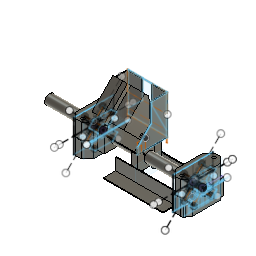
x-y-axis-on-pipe (Autodesk Fusion 360 design; units mm, degrees)
Autodesk Fusion 360 part; units mm, degrees
sketch "Sketch1" plane through (0, 0, 0) normal (1, 0, 0) x (0, 1, 0) in component "pipe-d25mm"
  circle A0 centre (0, 0) radius 12.5
  circle A1 centre (0, 0) radius 11
  dimension "d1" = 25
  dimension "d4" = 22
  constraint coincident A0.centre A1.centre
  constraint concentric A0 A1
  measures "d1" diameter of A0
  measures "d4" diameter of A1
extrude "Extrude1" add sketch "Sketch1" against normal blind 395 makes body 1 in component "pipe-d25mm"
sketch "Sketch1 (2)" plane through (0, 0, 0) normal (1, 0, 0) x (0, 1, 0) in component "pipe-slider"
  circle A0 centre (0, 0) radius 11
  circle A1 centre (0, 0) radius 12.5
  line L0 (0, 0) -> (50, 0) construction
  line L1 (50, 0) -> (50, -40) construction
  line L2 (50, -40) -> (0, -40) construction
  line L3 (0, -40) -> (0, 0) construction
  line L4 (50, 0) -> (-50, 0)
  line L5 (-50, 0) -> (-50, -40)
  line L6 (-50, -40) -> (50, -40)
  line L7 (50, -40) -> (50, 0)
  line L8 (0, 0) -> (61.3417, -61.3417) construction
  line L9 (0, 0) -> (86.7503, 0) construction
  line L10 (0, 0) -> (-70.1783, -70.1783) construction
  line L11 (0, 0) -> (99.2472, 0) construction
  line L12 (8.8388, -8.8388) -> (24.3952, -24.3952) construction
  line L13 (8.8388, -8.8388) -> (16.617, -16.617) construction
  line L14 (-8.8388, -8.8388) -> (-16.617, -16.617) construction
  line L15 (8.8388, -8.8388) -> (24.3952, -24.3952) construction
  line L16 (24.3952, -24.3952) -> (27.9307, -20.8597) construction
  line L17 (27.9307, -20.8597) -> (12.3744, -5.3033) construction
  line L18 (12.3744, -5.3033) -> (8.8388, -8.8388) construction
  line L19 (-8.8388, -8.8388) -> (-24.3952, -24.3952) construction
  line L20 (-24.3952, -24.3952) -> (-27.9307, -20.8597) construction
  line L21 (-27.9307, -20.8597) -> (-12.3744, -5.3033) construction
  line L22 (12.3744, -5.3033) -> (5.3033, -12.3744) construction
  line L23 (5.3033, -12.3744) -> (22.2739, -29.3449) construction
  line L24 (22.2739, -29.3449) -> (29.3449, -22.2739) construction
  line L25 (29.3449, -22.2739) -> (12.3744, -5.3033) construction
  line L26 (-5.3033, -12.3744) -> (-22.2739, -29.3449) construction
  line L27 (-22.2739, -29.3449) -> (-29.3449, -22.2739) construction
  line L28 (-29.3449, -22.2739) -> (-12.3744, -5.3033) construction
  line L29 (29.3449, -22.2739) -> (22.2739, -29.3449)
  line L30 (4, 0) -> (5.5355, 1.5355)
  circle A2 centre (0, 0) radius 13.5
  line L31 (22.2739, -29.3449) -> (5.3033, -12.3744)
  line L32 (12.3744, -5.3033) -> (29.3449, -22.2739)
  line L33 (-5.3033, -12.3744) -> (-22.2739, -29.3449)
  line L34 (-22.2739, -29.3449) -> (-29.3449, -22.2739)
  line L35 (-29.3449, -22.2739) -> (-12.3744, -5.3033)
  dimension "d5" = 50
  dimension "d6" = 40
  dimension "d7" = 100
  dimension "d8" = 45
  dimension "d9" = 135
  dimension "d10" = 22
  dimension "d11" = 11
  dimension "d12" = 11
  dimension "d13" = 5
  dimension "d14" = 22
  dimension "d15" = 5
  dimension "d16" = 10
  dimension "d17" = 24
  dimension "d18" = 10
  dimension "d19" = 24
  dimension "d20" = 27
  dimension "d21" = 24
  constraint horizontal L0
  constraint vertical L1
  constraint horizontal L2
  constraint vertical L3
  constraint coincident A0.centre A1.centre
  constraint horizontal L4
  constraint vertical L5
  constraint horizontal L6
  constraint vertical L7
  constraint horizontal L9
  constraint horizontal L11
  constraint coincident L8 L12.start
  constraint coincident A1 L12.start
  constraint parallel L8 L12
  constraint parallel L8 L13
  constraint coincident L10 L14.start
  constraint coincident A1 L14.start
  constraint perpendicular L13 L14
  constraint perpendicular L15 L16
  constraint parallel L15 L17
  constraint parallel L16 L18
  constraint perpendicular L19 L20
  constraint parallel L19 L21
  constraint coincident L10 L19.end
  constraint perpendicular L22 L23
  constraint parallel L22 L24
  constraint parallel L23 L25
  constraint perpendicular L12 L22
  constraint parallel L26 L28
  constraint perpendicular L29 L31
  constraint parallel L29 L30
  constraint coincident L0 L30.start
  constraint parallel L33 L35
  measures "d5" distance of A0.centre L0.end
  measures "d6" distance of A0.centre L2.end
  measures "d7" distance of L0.end L4.end
  measures "d8" angle of L8 L9
  measures "d9" angle of L10 L11
  measures "d10" distance of L12.start L12.end
  measures "d11" distance of L12.start L13.end
  measures "d12" distance of L14.start L14.end
  measures "d13" distance of L12.start L17.end
  measures "d14" distance of L14.start L19.end
  measures "d15" distance of L14.start L21.end
  measures "d16" distance of L17.end L22.end
  measures "d17" distance of L17.end L24.end
  measures "d18" distance of L21.end L26.start
  measures "d19" distance of L21.end L27.end
  measures "d20" diameter of A2
  measures "d21" distance of L21.end L27.end
extrude "Extrude7" add sketch "Sketch1 (2)" against normal blind 10 separate body contours L4 L5 L6 L7 L29 A2 L31 L32 L33 L34 L35 | L29 A2 L31 L32 | A2 L33 L34 L35 makes body 2 in component "pipe-slider"
extrude "Extrude1'" add sketch "Sketch1 (2)" along normal blind 24 separate body contours L4 L5 L6 L7 L29 A2 L31 L32 L33 L34 L35 makes body 3 in component "pipe-slider"
sketch "Sketch2" plane through (24, 0, 0) normal (1, 0, 0) x (0, 1, 0) in component "pipe-slider"
  line L0 (-5.3315, -12.4026) -> (-22.2739, -29.3449)
  line L1 (-22.2739, -29.3449) -> (-29.3449, -22.2739)
  line L2 (-29.3449, -22.2739) -> (-12.4026, -5.3315)
  arc A0 (-13.5, 0) -> (-12.4026, -5.3315) centre (0, 0) ccw
  line L3 (-13.5, 0) -> (-50, 0)
  line L4 (-50, 0) -> (-50, -40)
  line L5 (-50, -40) -> (50, -40)
  line L6 (50, -40) -> (50, 0)
  line L7 (50, 0) -> (13.5, 0)
  arc A1 (12.4026, -5.3315) -> (13.5, 0) centre (0, 0) ccw
  line L8 (12.4026, -5.3315) -> (29.3449, -22.2739)
  line L9 (29.3449, -22.2739) -> (22.2739, -29.3449)
  line L10 (22.2739, -29.3449) -> (5.3315, -12.4026)
  arc A2 (-5.3315, -12.4026) -> (5.3315, -12.4026) centre (0, 0) ccw
sketch "Sketch3" plane through (0, 3.5355, -3.5355) normal (0, -0.707107, 0.707107) x (1, 0, 0) in component "pipe-slider"
  line L0 (0, -12.5399) -> (0, -36.5)
  line L1 (0, -36.5) -> (24, -36.5)
  line L2 (24, -36.5) -> (24, -12.5399)
  line L3 (24, -12.5399) -> (0, -12.5399)
  line L4 (0, -36.5) -> (24, -36.5) construction
  line L5 (24, -36.5) -> (24, -34.5) construction
  line L6 (24, -34.5) -> (0, -34.5) construction
  line L7 (0, -34.5) -> (0, -36.5) construction
  line L8 (0, -34.5) -> (1, -34.5) construction
  line L9 (1, -34.5) -> (1, -12.5) construction
  line L10 (1, -12.5) -> (0, -12.5) construction
  line L11 (0, -12.5) -> (0, -34.5) construction
  line L12 (1, -34.5) -> (1, -12.5) construction
  line L13 (1, -12.5) -> (23, -12.5) construction
  line L14 (23, -12.5) -> (23, -34.5) construction
  line L15 (23, -34.5) -> (1, -34.5) construction
  line L16 (1, -34.5) -> (23, -12.5) construction
  line L17 (23, -34.5) -> (1, -12.5) construction
  circle A0 centre (12, -23.5) radius 4
  dimension "d24" = 2
  dimension "d25" = 22
  dimension "d26" = 22
  dimension "d27" = 22
  dimension "d28" = 8
  constraint perpendicular L4 L5
  constraint parallel L4 L6
  constraint parallel L5 L7
  constraint coincident L1.end L2.start
  constraint perpendicular L2 L4
  constraint coincident L0.end L1.start
  constraint perpendicular L8 L9
  constraint parallel L8 L10
  constraint parallel L9 L11
  constraint coincident L6 L8.end
  constraint perpendicular L12 L13
  constraint parallel L12 L14
  constraint parallel L13 L15
  constraint perpendicular L3 L12
  constraint midpoint L17 A0.centre
  measures "d24" distance of L0.end L6.end
  measures "d25" distance of L6.end L10.end
  measures "d26" distance of L8.end L9.end
  measures "d27" distance of L8.end L14.end
  measures "d28" diameter of A0
extrude "Extrude3" cut sketch "Sketch3" along normal blind 38 contours A0 bodies 3 in component "pipe-slider"
extrude "Extrude2" cut sketch "Sketch3" against normal blind 10 contours A0 bodies 3 in component "pipe-slider"
sketch "Sketch4" plane through (0, -3.5355, -3.5355) normal (0, 0.707107, 0.707107) x (-1, 0, 0) in component "pipe-slider"
  line L0 (0, -36.5) -> (0, -12.5399)
  line L1 (0, -12.5399) -> (-24, -12.5399)
  line L2 (-24, -12.5399) -> (-24, -36.5)
  line L3 (-24, -36.5) -> (0, -36.5)
  line L4 (0, -36.5) -> (-24, -36.5) construction
  line L5 (-24, -36.5) -> (-24, -34.5) construction
  line L6 (-24, -34.5) -> (0, -34.5) construction
  line L7 (0, -34.5) -> (0, -36.5) construction
  line L8 (-24, -34.5) -> (-23, -34.5) construction
  line L9 (-23, -34.5) -> (-23, -12.5) construction
  line L10 (-23, -12.5) -> (-24, -12.5) construction
  line L11 (-24, -12.5) -> (-24, -34.5) construction
  line L12 (-23, -34.5) -> (-1, -34.5) construction
  line L13 (-1, -34.5) -> (-1, -12.5) construction
  line L14 (-1, -12.5) -> (-23, -12.5) construction
  line L15 (-23, -12.5) -> (-23, -34.5) construction
  line L16 (-1, -34.5) -> (-23, -12.5) construction
  line L17 (-23, -34.5) -> (-1, -12.5) construction
  circle A0 centre (-12, -23.5) radius 4
  dimension "d33" = 2
  dimension "d34" = 22
  dimension "d35" = 22
  dimension "d36" = 8
  constraint perpendicular L4 L5
  constraint parallel L4 L6
  constraint parallel L5 L7
  constraint coincident L2.end L3.start
  constraint perpendicular L2 L4
  constraint coincident L0.start L3.end
  constraint perpendicular L8 L9
  constraint parallel L8 L10
  constraint parallel L9 L11
  constraint coincident L6 L8.end
  constraint perpendicular L2 L8
  constraint perpendicular L12 L13
  constraint parallel L12 L14
  constraint parallel L13 L15
  constraint coincident L6 L12.end
  constraint midpoint L17 A0.centre
  measures "d33" distance of L0.start L6.end
  measures "d34" distance of L5.end L10.end
  measures "d35" distance of L8.end L9.end
  measures "d36" diameter of A0
extrude "Extrude5" cut sketch "Sketch4" along normal blind 45 contours A0 bodies 3 in component "pipe-slider"
extrude "Extrude4" cut sketch "Sketch4" against normal blind 10 contours A0 bodies 3 in component "pipe-slider"
sketch "Sketch1 (3)" plane through (0, -3.5355, -3.5355) normal (0, 0.707107, 0.707107) x (-1, 0, 0) in component "washer"
  circle A0 centre (-12, -23.5) radius 3.5
  circle A1 centre (-12, -23.5) radius 8
  dimension "d41" = 7
  dimension "d42" = 16
  constraint concentric A0 A1
  measures "d41" diameter of A0
  measures "d42" diameter of A1
extrude "Extrude1''" add sketch "Sketch1 (3)" along normal blind 1.5 separate body makes body 4 in component "washer"
sketch "Sketch1 (4)" plane through (0, -2.4749, -2.4749) normal (0, 0.707107, 0.707107) x (-1, 0, 0) in component "bearing8x22x7"
  circle A0 centre (-12, -23.5) radius 3.5
  circle A1 centre (-12, -23.5) radius 8
  circle A2 centre (-12, -23.5) radius 3.5
  circle A3 centre (-12, -23.5) radius 11
  dimension "d45" = 22
  constraint concentric A0 A2
  constraint concentric A2 A3
  measures "d45" diameter of A3
extrude "Extrude1'''" add sketch "Sketch1 (4)" along normal blind 7 separate body contours A1 | A3 makes body 5 in component "bearing8x22x7"
sketch "Sketch6" plane through (24, 0, 0) normal (1, 0, 0) x (0, 1, 0) in component "pipe-slider"
  arc A0 (-13.5, 0) -> (13.5, 0) centre (0, 0) ccw
  line L0 (-13.5, 0) -> (-33.4897, -23.065)
  line L1 (-33.4897, -23.065) -> (-19.8622, -34.8755)
  line L2 (-19.8622, -34.8755) -> (24.3662, -35.2868)
  line L3 (24.3662, -35.2868) -> (35.669, -22.2451)
  line L4 (35.669, -22.2451) -> (13.5, 0)
  constraint coincident A0.centre origin
  constraint perpendicular L0 L1
  constraint perpendicular L1 L3
extrude "Extrude6" add sketch "Sketch2" sketch "Sketch6" along normal blind 10 of sketch 2 bodies 3 in component "pipe-slider"
sketch "Sketch7" plane through (0, 0, 0) normal (0, 0, 1) x (-1, 0, 0) in component "pipe-slider"
  ellipse E0 centre (-12, -33.234) end of major axis (-12, -27.5772) minor radius 4
  line L0 (0, -50) -> (0, -13.5)
  line L1 (0, -13.5) -> (-34, -13.5)
  line L2 (-34, -13.5) -> (-34, -50)
  line L3 (-34, -50) -> (0, -50)
  circle A0 centre (-12.5, -40) radius 4
  circle A1 centre (-12.5, 40) radius 4
  dimension "d52" = 8
  dimension "d53" = 8
  measures "d52" diameter of A0
  measures "d53" diameter of A1
extrude "Extrude8" cut sketch "Sketch7" against normal blind 46 contours E0 A0 | E0 A0 | A1 picked at (-12.249, -36.9652) picked at (-12.4627, -42.2784) bodies 3 in component "pipe-slider"
combine "Combine1" operation add target body 2 tool bodies 3 in component "pipe-slider"
chamfer "Chamfer1" distance 15 angle 45 4 edges at (34, 50, -20) (34, -50, -20) (-10, -50, -20) (-10, 50, -20) on bodies 2 in component "pipe-slider"
sketch "Sketch8" plane through (34, 0, 0) normal (1, 0, 0) x (0, 1, 0) in component "pipe-slider"
  line L0 (-35, 0) -> (-35, -40)
  line L1 (-35, -40) -> (35, -40)
  line L2 (35, -40) -> (35, 0)
  line L3 (35, 0) -> (13.5, 0)
  arc A0 (-13.5, 0) -> (13.5, 0) centre (0, 0) ccw
  line L4 (-13.5, 0) -> (-35, 0)
  line L5 (-52, 1) -> (-52, -0.5)
  line L6 (-52, 1) -> (55.5207, 1)
  line L7 (55.5207, 1) -> (55.5207, -0.5)
  line L8 (55.5207, -0.5) -> (-52, -0.5)
  line L9 (-52, -0.5) -> (-52, 1)
  dimension "d57" = 1.5
  constraint vertical L5
  constraint horizontal L6
  constraint vertical L7
  constraint horizontal L8
  constraint vertical L9
  measures "d57" distance of L5.start L5.end
extrude "Extrude9" cut sketch "Sketch8" against normal blind 61 contours L0 A0 L4 L8 | L0 L2 L3 A0 L4 L5 L6 L7 L8 L9 | L2 L3 A0 L8 bodies 2 in component "pipe-slider"
sketch "Sketch1 (5)" plane through (0, -10.6066, -10.6066) normal (0, 0.707107, 0.707107) x (-1, 0, 0) in component "stud-30mm-d8mm"
  circle A0 centre (-12, -23.5) radius 4
extrude "Extrude1''''" add sketch "Sketch1 (5)" along normal blind 30 separate body makes body 6 in component "stud-30mm-d8mm"
sketch "Sketch1 (6)" plane through (-10, 0, 0) normal (-1, 0, 0) x (0, -1, 0) in component "frame-bottom"
  line L0 (35, -0.5) -> (13.4907, -0.5)
  arc A0 (-13.4907, -0.5) -> (13.4907, -0.5) centre (0, 0) ccw
  line L1 (-13.4907, -0.5) -> (-35, -0.5)
  line L2 (-35, -0.5) -> (-35, -40)
  line L3 (-35, -40) -> (35, -40)
  line L4 (35, -40) -> (35, -0.5)
  line L5 (30, 20) -> (-45, 20)
  line L6 (-45, 20) -> (-45, 118)
  line L7 (-45, 118) -> (-4, 118)
  line L8 (30, 35) -> (30, 20)
  line L9 (-45, 118) -> (-4, 118) construction
  line L10 (-45, 70) -> (-45, 118) construction
  line L11 (30, 20) -> (20, 20) construction
  line L12 (20, 20) -> (20, 35) construction
  line L13 (20, 35) -> (30, 35) construction
  line L14 (30, 35) -> (30, 20) construction
  line L15 (30, 35) -> (-4, 70)
  line L16 (-4, 118) -> (-4, 70)
  line L17 (30, 20) -> (10, 20) construction
  line L18 (10, 20) -> (10, 46) construction
  line L19 (10, 46) -> (30, 46) construction
  line L20 (30, 46) -> (30, 20) construction
  circle A1 centre (10, 46) radius 4
  dimension "d66" = 75
  dimension "d68" = 41
  dimension "d69" = 48
  dimension "d98" = 26
  dimension "d99" = 8
  constraint horizontal L5
  constraint vertical L6
  constraint horizontal L7
  constraint vertical L8
  constraint horizontal L9
  constraint vertical L10
  constraint horizontal L11
  constraint vertical L12
  constraint horizontal L13
  constraint vertical L14
  constraint perpendicular L7 L16
  constraint horizontal L17
  constraint vertical L18
  constraint horizontal L19
  constraint vertical L20
  constraint coincident L18.end L19.start
  measures "d66" distance of L5.start L5.end
  measures "d68" distance of L6.end L7.end
  measures "d69" distance of L6.end L10.start
  measures "d98" distance of L5.start L19.end
  measures "d99" diameter of A1
extrude "Extrude1'''''" add sketch "Sketch1 (6)" along normal blind 100 separate body contours L5 L6 L7 L8 L15 L16 makes body 7 in component "frame-bottom"
sketch "Sketch5" plane through (0, 45, 0) normal (0, 1, 0) x (-1, 0, 0) in component "frame-bottom"
  line L0 (10, 118) -> (12, 118) construction
  line L1 (12, 118) -> (12, 8) construction
  line L2 (12, 8) -> (10, 8) construction
  line L3 (10, 8) -> (10, 118) construction
  line L4 (110, 118) -> (108, 118) construction
  line L5 (108, 118) -> (108, 8) construction
  line L6 (108, 8) -> (110, 8) construction
  line L7 (110, 8) -> (110, 118) construction
  line L8 (110, 20) -> (10, 20) construction
  line L9 (10, 20) -> (10, 22) construction
  line L10 (10, 22) -> (110, 22) construction
  line L11 (110, 22) -> (110, 20) construction
  line L12 (12, 118) -> (108, 118) construction
  line L13 (108, 118) -> (108, 22) construction
  line L14 (108, 22) -> (12, 22) construction
  line L15 (12, 22) -> (12, 118) construction
  line L16 (12, 118) -> (108, 118)
  line L17 (108, 118) -> (108, 22)
  line L18 (108, 22) -> (12, 22)
  line L19 (12, 22) -> (12, 118)
  line L20 (10, 118) -> (110, 118) construction
  line L21 (110, 118) -> (110, 70) construction
  line L22 (110, 70) -> (10, 70) construction
  line L23 (10, 70) -> (10, 118) construction
  line L24 (10, 20) -> (110, 20) construction
  line L25 (110, 20) -> (110, 35) construction
  line L26 (110, 35) -> (10, 35) construction
  line L27 (10, 35) -> (10, 20) construction
  line L28 (10, 118) -> (48, 118) construction
  line L29 (48, 118) -> (48, 70) construction
  line L30 (48, 70) -> (10, 70) construction
  line L31 (10, 70) -> (10, 118) construction
  line L32 (110, 118) -> (72, 118) construction
  line L33 (72, 118) -> (72, 70) construction
  line L34 (72, 70) -> (110, 70) construction
  line L35 (110, 70) -> (110, 118) construction
  line L36 (48, 118) -> (48, 70)
  line L37 (48, 70) -> (12, 35)
  line L38 (108, 118) -> (72, 118)
  line L39 (72, 70) -> (72, 118)
  line L40 (72, 70) -> (108, 35)
  dimension "d81" = 110
  dimension "d82" = 2
  dimension "d83" = 110
  dimension "d84" = 100
  dimension "d85" = 2
  dimension "d90" = 48
  dimension "d91" = 15
  dimension "d92" = 38
  dimension "d93" = 38
  constraint horizontal L0
  constraint vertical L1
  constraint horizontal L2
  constraint vertical L3
  constraint horizontal L4
  constraint vertical L5
  constraint horizontal L6
  constraint vertical L7
  constraint horizontal L8
  constraint vertical L9
  constraint horizontal L10
  constraint vertical L11
  constraint coincident L7 L8.start
  constraint horizontal L12
  constraint vertical L13
  constraint horizontal L14
  constraint vertical L15
  constraint coincident L5 L13.end
  constraint coincident L10 L13.end
  constraint horizontal L16
  constraint vertical L17
  constraint horizontal L18
  constraint vertical L19
  constraint horizontal L20
  constraint vertical L21
  constraint horizontal L22
  constraint vertical L23
  constraint horizontal L24
  constraint vertical L25
  constraint horizontal L26
  constraint vertical L27
  constraint horizontal L28
  constraint vertical L29
  constraint horizontal L30
  constraint vertical L31
  constraint horizontal L32
  constraint vertical L33
  constraint horizontal L34
  constraint vertical L35
  constraint coincident L15 L37.end
  constraint coincident L26 L37.end
  constraint coincident L13 L40.end
  constraint coincident L26 L40.end
  measures "d81" distance of L0.start L2.end
  measures "d82" distance of L4.start L4.end
  measures "d83" distance of L4.start L6.end
  measures "d84" distance of L8.start L8.end
  measures "d85" distance of L8.start L10.end
  measures "d90" distance of L0.start L22.end
  measures "d91" distance of L8.end L26.end
  measures "d92" distance of L0.start L28.end
  measures "d93" distance of L4.start L32.end
extrude "Extrude5'" add sketch "Sketch5" against normal blind 2 contours L16 L19 L36 L37 | L16 L17 L38 L39 L40 bodies 7 in component "frame-bottom"
extrude "Extrude4'" cut sketch "Sketch5" against normal blind 120 bodies 7 in component "frame-bottom"
extrude "Extrude6'" add sketch "Sketch5" against normal blind 2 contours L16 L19 L36 L37 | L16 L17 L38 L39 L40 bodies 7 in component "frame-bottom"
sketch "Sketch1 (7)" plane through (-10, 0, 0) normal (-1, 0, 0) x (0, -1, 0) in component "frame-top"
  line L0 (30, 20) -> (-45, 20)
  line L1 (-45, 20) -> (-45, 96)
  line L2 (-45, 96) -> (-4, 96)
  line L3 (-4, 96) -> (-4, 70)
  line L4 (-4, 70) -> (30, 35)
  line L5 (30, 35) -> (30, 20)
  line L6 (-45, 96) -> (-38, 96) construction
  line L7 (-38, 96) -> (-38, 76) construction
  line L8 (-38, 76) -> (-45, 76) construction
  line L9 (-45, 76) -> (-45, 96) construction
  circle A0 centre (-38, 76) radius 4
  dimension "d101" = 76
  dimension "d112" = 7
  dimension "d113" = 20
  dimension "d114" = 8
  constraint horizontal L0
  constraint perpendicular L0 L1
  constraint perpendicular L1 L2
  constraint perpendicular L2 L3
  constraint horizontal L6
  constraint vertical L7
  constraint horizontal L8
  constraint vertical L9
  constraint coincident L7.end L8.start
  measures "d101" distance of L0.end L1.end
  measures "d112" distance of L1.end L6.end
  measures "d113" distance of L1.end L8.end
  measures "d114" diameter of A0
extrude "Extrude2'" add sketch "Sketch1 (7)" along normal blind 80 separate body makes body 8 in component "frame-top"
sketch "Sketch2 (2)" plane through (0, 45, 0) normal (0, 1, 0) x (-1, 0, 0) in component "frame-top"
  line L0 (10, 96) -> (10, 20)
  line L1 (10, 20) -> (90, 20)
  line L2 (90, 20) -> (90, 96)
  line L3 (90, 96) -> (10, 96)
  line L4 (12, 97) -> (88, 97)
  line L5 (88, 97) -> (88, 22)
  line L6 (88, 22) -> (12, 22)
  line L7 (12, 22) -> (12, 97)
  constraint horizontal L4
  constraint vertical L5
  constraint horizontal L6
  constraint vertical L7
extrude "Extrude3'" cut sketch "Sketch2 (2)" against normal blind 156 contours L3 L5 L6 L7 bodies 8 in component "frame-top"
sketch "Sketch3 (2)" plane through (0, 45, 0) normal (0, 1, 0) x (-1, 0, 0) in component "frame-top"
  line L0 (88, 96) -> (88, 22)
  line L1 (88, 22) -> (12, 22)
  line L2 (12, 22) -> (12, 96)
  line L3 (12, 96) -> (10, 96)
  line L4 (10, 96) -> (10, 20)
  line L5 (10, 20) -> (90, 20)
  line L6 (90, 20) -> (90, 96)
  line L7 (90, 96) -> (88, 96)
  line L8 (10, 96) -> (90, 96) construction
  line L9 (90, 96) -> (90, 70) construction
  line L10 (90, 70) -> (10, 70) construction
  line L11 (10, 70) -> (10, 96) construction
  line L12 (10, 96) -> (48, 96)
  line L13 (48, 96) -> (48, 70)
  line L14 (48, 70) -> (12, 35)
  line L15 (12, 35) -> (10, 35)
  line L16 (90, 96) -> (52, 96)
  line L17 (52, 96) -> (52, 70)
  line L18 (52, 70) -> (88, 35)
  line L19 (88, 35) -> (90, 35)
  dimension "d108" = 26
  dimension "d109" = 38
  constraint horizontal L8
  constraint vertical L9
  constraint horizontal L10
  constraint vertical L11
  constraint coincident L3.end L4.start
  constraint coincident L8 L12.end
  constraint coincident L10 L13.end
  constraint perpendicular L10 L13
  constraint coincident L2 L14.end
  constraint coincident L4 L15.end
  constraint perpendicular L4 L15
  constraint coincident L6.end L7.start
  constraint coincident L8 L16.end
  constraint perpendicular L9 L16
  constraint coincident L10 L17.end
  constraint perpendicular L10 L17
  constraint coincident L0 L18.end
  constraint coincident L6 L19.end
  constraint perpendicular L6 L19
  measures "d108" distance of L3.end L10.end
  measures "d109" distance of L3.end L12.end
extrude "Extrude4''" add sketch "Sketch3 (2)" against normal blind 2 contours L0 L16 L17 L18 | L2 L12 L13 L14 bodies 8 in component "frame-top"
sketch "Sketch1 (8)" plane through (0, -66, 0) normal (0, -1, 0) x (1, 0, 0) in component "cut-tool-12x12"
  line L0 (-120, 39) -> (-120, 114)
  line L1 (-120, 114) -> (-200, 114)
  line L2 (-200, 114) -> (-200, 39)
  line L3 (-200, 39) -> (-120, 39)
  line L4 (-155, 15) -> (-161, 15)
  line L5 (-167, 20.9289) -> (-167, 115)
  line L6 (-167, 115) -> (-155, 115)
  line L7 (-155, 115) -> (-155, 31)
  line L8 (-161, 15) -> (-167, 20.9289)
  line L9 (-155, 15) -> (-150, 15)
  line L10 (-150, 15) -> (-154, 30)
  line L11 (-154, 30) -> (-155, 31)
  constraint horizontal L4
  constraint vertical L5
  constraint horizontal L6
  constraint vertical L7
  constraint perpendicular L7 L9
extrude "Extrude1''''''" add sketch "Sketch1 (8)" along normal blind 12 separate body contours L3 L4 L5 L7 L8 L9 L10 L11 | L1 L3 L5 L7 makes body 9 in component "cut-tool-12x12"
sketch "Sketch1 (9)" plane through (-10, 0, 0) normal (-1, 0, 0) x (0, -1, 0) in component "pipe-to-frame-clump"
  line L0 (35, -0.5) -> (13.4907, -0.5)
  arc A0 (-13.4907, -0.5) -> (13.4907, -0.5) centre (0, 0) ccw
  line L1 (-13.4907, -0.5) -> (-35, -0.5)
  line L2 (-35, -0.5) -> (-35, -40)
  line L3 (-35, -40) -> (35, -40)
  line L4 (35, -40) -> (35, -0.5)
  line L5 (-30, 19) -> (-30, -16)
  line L6 (-30, -21) -> (30, -21)
  line L7 (30, -21) -> (30, 19)
  line L8 (30, 19) -> (14, 19)
  line L9 (-30, 19) -> (-14, 19)
  arc A1 (-12.4631, -0.9597) -> (12.4631, -0.9597) centre (0, 0) ccw
  line L10 (-14, 19) -> (-12.4631, -0.9597)
  line L11 (14, 19) -> (12.4631, -0.9597)
  line L12 (-30, -16) -> (-30, -21)
  dimension "d123" = 12.5
  constraint vertical L5
  constraint perpendicular L5 L6
  constraint perpendicular L6 L7
  constraint perpendicular L7 L8
  constraint perpendicular L5 L9
  constraint coincident A0.centre A1.centre
  constraint tangent A1 L10
  constraint tangent A1 L11
  constraint parallel L5 L12
  measures "d123" radius of A1
extrude "Extrude1'''''''" add sketch "Sketch1 (9)" along normal blind 16 separate body contours L0 A0 L1 L5 L6 L7 L12 | L0 A0 L1 L5 L7 L8 L9 A1 L10 L11 makes body 10 in component "pipe-to-frame-clump"
sketch "Sketch2 (3)" plane through (0, 0, -21) normal (0, 0, -1) x (1, 0, 0) in component "pipe-to-frame-clump"
  line L0 (-10, -30) -> (-10, 30)
  line L1 (-10, 30) -> (-26, 30)
  line L2 (-26, 30) -> (-26, -30)
  line L3 (-26, -30) -> (-10, -30)
  line L4 (-26, 30) -> (-18, 30) construction
  line L5 (-18, 30) -> (-18, 22) construction
  line L6 (-18, 22) -> (-26, 22) construction
  line L7 (-26, 22) -> (-26, 30) construction
  line L8 (-10, -30) -> (-18, -30) construction
  line L9 (-18, -30) -> (-18, -22) construction
  line L10 (-18, -22) -> (-10, -22) construction
  line L11 (-10, -22) -> (-10, -30) construction
  circle A0 centre (-18, 22) radius 4
  circle A1 centre (-18, -22) radius 4
  dimension "d126" = 8
  dimension "d127" = 8
  dimension "d128" = 8
  dimension "d129" = 8
  constraint horizontal L4
  constraint vertical L5
  constraint horizontal L6
  constraint vertical L7
  constraint coincident L1.end L2.start
  constraint horizontal L8
  constraint vertical L9
  constraint horizontal L10
  constraint vertical L11
  constraint coincident L0.start L3.end
  constraint coincident L5.end L6.start
  constraint coincident L9.end L10.start
  measures "d126" distance of L1.end L6.end
  measures "d127" distance of L0.start L10.end
  measures "d128" diameter of A0
  measures "d129" diameter of A1
extrude "Extrude7'" cut sketch "Sketch2 (3)" against normal blind 50 contours A0 | A1 bodies 7 in component "frame-bottom"
extrude "Extrude2''" cut sketch "Sketch2 (3)" against normal blind 50 contours A0 | A1 bodies 10 in component "pipe-to-frame-clump"
sketch "Sketch1 (10)" plane through (-110, 0, 0) normal (1, 0, 0) x (0, 1, 0) in component "pipe-to-frame-clump-insert"
  line L0 (30, -21) -> (30, 19)
  line L1 (30, 19) -> (14, 19)
  line L2 (14, 19) -> (12.4631, -0.9597)
  arc A0 (-12.4631, -0.9597) -> (12.4631, -0.9597) centre (0, 0) ccw
  line L3 (-12.4631, -0.9597) -> (-14, 19)
  line L4 (-14, 19) -> (-30, 19)
  line L5 (-30, 19) -> (-30, -21)
  line L6 (-30, -21) -> (30, -21)
  arc A1 (12.4494, 2.9753) -> (-12.4379, 3.0232) centre (0, 0) ccw
  line L7 (-12.4379, 3.0232) -> (-13.7428, 19.9704)
  line L8 (12.4494, 2.9753) -> (13.7582, 19.972)
  line L9 (13.7582, 19.972) -> (-13.7428, 19.9704)
  dimension "d134" = 12.8
  constraint coincident A0.centre A1.centre
  constraint parallel L3 L7
  constraint parallel L2 L8
  measures "d134" radius of A1
extrude "Extrude1''''''''" add sketch "Sketch1 (10)" against normal up to surface (16 mm away) separate body contours A1 L7 L8 L9 makes body 11 in component "pipe-to-frame-clump-insert"
sketch "Sketch1 (11)" plane through (0, 0, -29.5) normal (0, 0, -1) x (1, 0, 0) in component "nut-m8"
  circle A0 centre (-118, 22) radius 3.5
  circle A1 centre (-118, 22) radius 11
  line L0 (-111.5327, 18.1912) -> (-111.4678, 25.6965)
  line L1 (-111.4678, 25.6965) -> (-117.9352, 29.5053)
  line L2 (-117.9352, 29.5053) -> (-124.4673, 25.8088)
  line L3 (-124.4673, 25.8088) -> (-124.5322, 18.3035)
  line L4 (-124.5322, 18.3035) -> (-118.0648, 14.4947)
  line L5 (-118.0648, 14.4947) -> (-111.5327, 18.1912)
  circle A2 centre (-118, 22) radius 4
  point P0 (-118, 22)
  dimension "d137" = 6.5
  dimension "d138" = 8
  constraint coincident P0 A0.centre
  measures "d137" distance of P0 L5
  measures "d138" diameter of A2
extrude "Extrude1'''''''''" add sketch "Sketch1 (11)" along normal blind 6.5 separate body contours L0 L1 L2 L3 L4 L5 makes body 12 in component "nut-m8"
sketch "Sketch1 (12)" plane through (-110, 0, 0) normal (-1, 0, 0) x (0, -1, 0) in component "corner"
  line L0 (65.5, -40) -> (33, -40)
  line L1 (33, -40) -> (33, -8)
  line L2 (33, -8) -> (35, -8)
  line L3 (35, -8) -> (35, -38)
  line L4 (35, -38) -> (65.5, -38)
  line L5 (65.5, -38) -> (65.5, -40)
  constraint horizontal L0
  constraint perpendicular L0 L1
  constraint perpendicular L1 L2
  constraint perpendicular L0 L3
  constraint perpendicular L3 L4
  constraint perpendicular L4 L5
extrude "Extrude1''''''''''" add sketch "Sketch1 (12)" along normal blind 150 separate body makes body 13 in component "corner"
sketch "Sketch1 (13)" plane through (0, 0, 0) normal (1, 0, 0) x (0, 1, 0) in component "pipe-slider2"
  circle A0 centre (0, 0) radius 11
  circle A1 centre (0, 0) radius 12.5
  line L0 (0, 0) -> (50, 0) construction
  line L1 (50, 0) -> (50, -40) construction
  line L2 (50, -40) -> (0, -40) construction
  line L3 (0, -40) -> (0, 0) construction
  line L4 (50, 0) -> (-50, 0)
  line L5 (-50, 0) -> (-50, -40)
  line L6 (-50, -40) -> (50, -40)
  line L7 (50, -40) -> (50, 0)
  line L8 (0, 0) -> (61.3417, -61.3417) construction
  line L9 (0, 0) -> (86.7503, 0) construction
  line L10 (0, 0) -> (-70.1783, -70.1783) construction
  line L11 (0, 0) -> (99.2472, 0) construction
  line L12 (8.8388, -8.8388) -> (24.3952, -24.3952) construction
  line L13 (8.8388, -8.8388) -> (16.617, -16.617) construction
  line L14 (-8.8388, -8.8388) -> (-16.617, -16.617) construction
  line L15 (8.8388, -8.8388) -> (24.3952, -24.3952) construction
  line L16 (24.3952, -24.3952) -> (27.9307, -20.8597) construction
  line L17 (27.9307, -20.8597) -> (12.3744, -5.3033) construction
  line L18 (12.3744, -5.3033) -> (8.8388, -8.8388) construction
  line L19 (-8.8388, -8.8388) -> (-24.3952, -24.3952) construction
  line L20 (-24.3952, -24.3952) -> (-27.9307, -20.8597) construction
  line L21 (-27.9307, -20.8597) -> (-12.3744, -5.3033) construction
  line L22 (12.3744, -5.3033) -> (5.3033, -12.3744) construction
  line L23 (5.3033, -12.3744) -> (22.2739, -29.3449) construction
  line L24 (22.2739, -29.3449) -> (29.3449, -22.2739) construction
  line L25 (29.3449, -22.2739) -> (12.3744, -5.3033) construction
  line L26 (-5.3033, -12.3744) -> (-22.2739, -29.3449) construction
  line L27 (-22.2739, -29.3449) -> (-29.3449, -22.2739) construction
  line L28 (-29.3449, -22.2739) -> (-12.3744, -5.3033) construction
  line L29 (29.3449, -22.2739) -> (22.2739, -29.3449)
  line L30 (4, 0) -> (5.5355, 1.5355)
  circle A2 centre (0, 0) radius 13.5
  line L31 (22.2739, -29.3449) -> (5.3033, -12.3744)
  line L32 (12.3744, -5.3033) -> (29.3449, -22.2739)
  line L33 (-5.3033, -12.3744) -> (-22.2739, -29.3449)
  line L34 (-22.2739, -29.3449) -> (-29.3449, -22.2739)
  line L35 (-29.3449, -22.2739) -> (-12.3744, -5.3033)
  line L36 (4, -17) -> (25.2311, -39.4799)
  line L37 (25.2311, -39.4799) -> (2, -39.4799)
  line L38 (2, -39.4799) -> (2, -19)
  line L39 (2, -19) -> (4, -17)
  line L40 (-2, -19) -> (-4, -17)
  line L41 (-4, -17) -> (-26.4799, -39.4799)
  line L42 (-26.4799, -39.4799) -> (-2, -39.4799)
  line L43 (-2, -39.4799) -> (-2, -19)
  line L44 (35, -10) -> (35, -39.5461)
  line L45 (45, -39.5461) -> (45, -10)
  line L46 (45, -39.5461) -> (35, -39.5461)
  line L47 (-45, -10) -> (-45, -39.4799)
  line L48 (-45, -39.4799) -> (-35, -39.4799)
  line L49 (-35, -10) -> (-35, -39.4799)
  line L50 (40, -5) -> (45, -10)
  line L51 (40, -5) -> (35, -10)
  line L52 (-35, -10) -> (-40, -5)
  line L53 (-45, -10) -> (-40, -5)
  line L54 (32, -39.5) -> (32, -25)
  line L55 (32, -25) -> (24.7291, -32.2709)
  line L56 (24.7291, -32.2709) -> (32, -39.5)
  line L57 (14.9682, -39.4799) -> (14.9682, -28.6134)
  line L58 (10.9999, -24.4117) -> (10.9999, -39.4799)
  line L59 (-15.9985, -39.4799) -> (-15.9985, -28.9985)
  line L60 (-11.6082, -24.6082) -> (-11.6082, -39.4799)
  line L61 (-31.9198, -39.3754) -> (-31.9198, -25.3181)
  line L62 (-31.9198, -25.3181) -> (-24.9, -32.7)
  line L63 (-24.9, -32.7) -> (-31.9198, -39.3754)
  dimension "d5_1" = 50
  dimension "d6_1" = 40
  dimension "d7_1" = 100
  dimension "d8_1" = 45
  dimension "d9_1" = 135
  dimension "d10_1" = 22
  dimension "d11_1" = 11
  dimension "d12_1" = 11
  dimension "d13_1" = 5
  dimension "d14_1" = 22
  dimension "d15_1" = 5
  dimension "d16_1" = 10
  dimension "d17_1" = 24
  dimension "d18_1" = 10
  dimension "d19_1" = 24
  dimension "d20_1" = 27
  dimension "d21_1" = 24
  constraint horizontal L0
  constraint vertical L1
  constraint horizontal L2
  constraint vertical L3
  constraint coincident A0.centre A1.centre
  constraint horizontal L4
  constraint vertical L5
  constraint horizontal L6
  constraint vertical L7
  constraint horizontal L9
  constraint horizontal L11
  constraint coincident L8 L12.start
  constraint coincident A1 L12.start
  constraint parallel L8 L12
  constraint parallel L8 L13
  constraint coincident L10 L14.start
  constraint coincident A1 L14.start
  constraint perpendicular L13 L14
  constraint perpendicular L15 L16
  constraint parallel L15 L17
  constraint parallel L16 L18
  constraint perpendicular L19 L20
  constraint parallel L19 L21
  constraint coincident L10 L19.end
  constraint perpendicular L22 L23
  constraint parallel L22 L24
  constraint parallel L23 L25
  constraint perpendicular L12 L22
  constraint parallel L26 L28
  constraint perpendicular L29 L31
  constraint parallel L29 L30
  constraint coincident L0 L30.start
  constraint parallel L33 L35
  constraint horizontal L37
  constraint perpendicular L37 L38
  constraint perpendicular L39 L40
  constraint perpendicular L40 L41
  constraint perpendicular L3 L42
  constraint perpendicular L42 L43
  constraint perpendicular L44 L46
  constraint perpendicular L46 L47
  constraint perpendicular L47 L48
  constraint perpendicular L48 L49
  constraint perpendicular L50 L51
  constraint perpendicular L52 L53
  constraint vertical L54
  constraint perpendicular L8 L55
  constraint coincident L37 L57.start
  constraint coincident L36 L57.end
  constraint perpendicular L37 L57
  constraint coincident L36 L58.start
  constraint coincident L37 L58.end
  constraint perpendicular L37 L58
  constraint coincident L42 L59.start
  constraint coincident L41 L59.end
  constraint perpendicular L42 L59
  constraint coincident L41 L60.start
  constraint coincident L42 L60.end
  constraint perpendicular L42 L60
  constraint perpendicular L6 L61
  constraint perpendicular L62 L63
  measures "d5_1" distance of A0.centre L0.end
  measures "d6_1" distance of A0.centre L2.end
  measures "d7_1" distance of L0.end L4.end
  measures "d8_1" angle of L8 L9
  measures "d9_1" angle of L10 L11
  measures "d10_1" distance of L12.start L12.end
  measures "d11_1" distance of L12.start L13.end
  measures "d12_1" distance of L14.start L14.end
  measures "d13_1" distance of L12.start L17.end
  measures "d14_1" distance of L14.start L19.end
  measures "d15_1" distance of L14.start L21.end
  measures "d16_1" distance of L17.end L22.end
  measures "d17_1" distance of L17.end L24.end
  measures "d18_1" distance of L21.end L26.start
  measures "d19_1" distance of L21.end L27.end
  measures "d20_1" diameter of A2
  measures "d21_1" distance of L21.end L27.end
extrude "Extrude1'''''''''''" add sketch "Sketch1 (13)" along normal blind 24 separate body contours L4 L5 L6 L7 L29 A2 L31 L32 L33 L34 L35 | L36 L37 L38 L39 L58 | L36 L37 L57 L58 | L36 L37 L57 | L40 L41 L42 L43 L60 | L41 L42 L59 L60 | L41 L42 L59 | L44 L45 L46 L50 L51 | L47 L48 L49 L52 L53 | L54 L55 L56 | L61 L62 L63 makes body 14 in component "pipe-slider2"
sketch "Sketch2 (4)" plane through (24, 0, 0) normal (1, 0, 0) x (0, 1, 0) in component "pipe-slider2"
  line L0 (-5.3315, -12.4026) -> (-22.2739, -29.3449)
  line L1 (-22.2739, -29.3449) -> (-29.3449, -22.2739)
  line L2 (-29.3449, -22.2739) -> (-12.4026, -5.3315)
  arc A0 (-13.5, 0) -> (-12.4026, -5.3315) centre (0, 0) ccw
  line L3 (-13.5, 0) -> (-50, 0)
  line L4 (-50, 0) -> (-50, -40)
  line L5 (-50, -40) -> (50, -40)
  line L6 (50, -40) -> (50, 0)
  line L7 (50, 0) -> (13.5, 0)
  arc A1 (12.4026, -5.3315) -> (13.5, 0) centre (0, 0) ccw
  line L8 (12.4026, -5.3315) -> (29.3449, -22.2739)
  line L9 (29.3449, -22.2739) -> (22.2739, -29.3449)
  line L10 (22.2739, -29.3449) -> (5.3315, -12.4026)
  arc A2 (-5.3315, -12.4026) -> (5.3315, -12.4026) centre (0, 0) ccw
sketch "Sketch3 (3)" plane through (0, 3.5355, -3.5355) normal (0, -0.707107, 0.707107) x (1, 0, 0) in component "pipe-slider2"
  line L0 (0, -12.5399) -> (0, -36.5)
  line L1 (0, -36.5) -> (24, -36.5)
  line L2 (24, -36.5) -> (24, -12.5399)
  line L3 (24, -12.5399) -> (0, -12.5399)
  line L4 (0, -36.5) -> (24, -36.5) construction
  line L5 (24, -36.5) -> (24, -34.5) construction
  line L6 (24, -34.5) -> (0, -34.5) construction
  line L7 (0, -34.5) -> (0, -36.5) construction
  line L8 (0, -34.5) -> (1, -34.5) construction
  line L9 (1, -34.5) -> (1, -12.5) construction
  line L10 (1, -12.5) -> (0, -12.5) construction
  line L11 (0, -12.5) -> (0, -34.5) construction
  line L12 (1, -34.5) -> (1, -12.5) construction
  line L13 (1, -12.5) -> (23, -12.5) construction
  line L14 (23, -12.5) -> (23, -34.5) construction
  line L15 (23, -34.5) -> (1, -34.5) construction
  line L16 (1, -34.5) -> (23, -12.5) construction
  line L17 (23, -34.5) -> (1, -12.5) construction
  circle A0 centre (12, -23.5) radius 4
  dimension "d24_1" = 2
  dimension "d25_1" = 22
  dimension "d26_1" = 22
  dimension "d27_1" = 22
  dimension "d28_1" = 8
  constraint perpendicular L4 L5
  constraint parallel L4 L6
  constraint parallel L5 L7
  constraint coincident L1.end L2.start
  constraint perpendicular L2 L4
  constraint coincident L0.end L1.start
  constraint perpendicular L8 L9
  constraint parallel L8 L10
  constraint parallel L9 L11
  constraint coincident L6 L8.end
  constraint perpendicular L12 L13
  constraint parallel L12 L14
  constraint parallel L13 L15
  constraint perpendicular L3 L12
  constraint midpoint L17 A0.centre
  measures "d24_1" distance of L0.end L6.end
  measures "d25_1" distance of L6.end L10.end
  measures "d26_1" distance of L8.end L9.end
  measures "d27_1" distance of L8.end L14.end
  measures "d28_1" diameter of A0
extrude "Extrude3''" cut sketch "Sketch3 (3)" along normal blind 38 contours A0 bodies 14 in component "pipe-slider2"
extrude "Extrude2'''" cut sketch "Sketch3 (3)" against normal blind 10 contours A0 bodies 14 in component "pipe-slider2"
sketch "Sketch4 (2)" plane through (0, -3.5355, -3.5355) normal (0, 0.707107, 0.707107) x (-1, 0, 0) in component "pipe-slider2"
  line L0 (0, -36.5) -> (0, -12.5399)
  line L1 (0, -12.5399) -> (-24, -12.5399)
  line L2 (-24, -12.5399) -> (-24, -36.5)
  line L3 (-24, -36.5) -> (0, -36.5)
  line L4 (0, -36.5) -> (-24, -36.5) construction
  line L5 (-24, -36.5) -> (-24, -34.5) construction
  line L6 (-24, -34.5) -> (0, -34.5) construction
  line L7 (0, -34.5) -> (0, -36.5) construction
  line L8 (-24, -34.5) -> (-23, -34.5) construction
  line L9 (-23, -34.5) -> (-23, -12.5) construction
  line L10 (-23, -12.5) -> (-24, -12.5) construction
  line L11 (-24, -12.5) -> (-24, -34.5) construction
  line L12 (-23, -34.5) -> (-1, -34.5) construction
  line L13 (-1, -34.5) -> (-1, -12.5) construction
  line L14 (-1, -12.5) -> (-23, -12.5) construction
  line L15 (-23, -12.5) -> (-23, -34.5) construction
  line L16 (-1, -34.5) -> (-23, -12.5) construction
  line L17 (-23, -34.5) -> (-1, -12.5) construction
  circle A0 centre (-12, -23.5) radius 4
  dimension "d33_1" = 2
  dimension "d34_1" = 22
  dimension "d35_1" = 22
  dimension "d36_1" = 8
  constraint perpendicular L4 L5
  constraint parallel L4 L6
  constraint parallel L5 L7
  constraint coincident L2.end L3.start
  constraint perpendicular L2 L4
  constraint coincident L0.start L3.end
  constraint perpendicular L8 L9
  constraint parallel L8 L10
  constraint parallel L9 L11
  constraint coincident L6 L8.end
  constraint perpendicular L2 L8
  constraint perpendicular L12 L13
  constraint parallel L12 L14
  constraint parallel L13 L15
  constraint coincident L6 L12.end
  constraint midpoint L17 A0.centre
  measures "d33_1" distance of L0.start L6.end
  measures "d34_1" distance of L5.end L10.end
  measures "d35_1" distance of L8.end L9.end
  measures "d36_1" diameter of A0
extrude "Extrude5''" cut sketch "Sketch4 (2)" along normal blind 45 contours A0 bodies 14 in component "pipe-slider2"
extrude "Extrude4'''" cut sketch "Sketch4 (2)" against normal blind 10 contours A0 bodies 14 in component "pipe-slider2"
sketch "Sketch6 (2)" plane through (24, 0, 0) normal (1, 0, 0) x (0, 1, 0) in component "pipe-slider2"
  arc A0 (-13.5, 0) -> (13.5, 0) centre (0, 0) ccw
  line L0 (-13.5, 0) -> (-33.4897, -23.065)
  line L1 (-33.4897, -23.065) -> (-19.8622, -34.8755)
  line L2 (-19.8622, -34.8755) -> (24.3662, -35.2868)
  line L3 (24.3662, -35.2868) -> (35.669, -22.2451)
  line L4 (35.669, -22.2451) -> (13.5, 0)
  constraint coincident A0.centre origin
  constraint perpendicular L0 L1
  constraint perpendicular L1 L3
sketch "Sketch7 (2)" plane through (0, 0, 0) normal (0, 0, 1) x (-1, 0, 0) in component "pipe-slider2"
  ellipse E0 centre (-12, -33.234) end of major axis (-12, -27.5772) minor radius 4
  line L0 (0, -50) -> (0, -13.5)
  line L1 (0, -13.5) -> (-24, -13.5)
  line L2 (-24, -50) -> (0, -50)
  circle A0 centre (-12.5, -40) radius 4
  circle A1 centre (-12.5, 40) radius 4
  line L3 (-24, -13.5) -> (-24, -50)
  dimension "d52_1" = 8
  dimension "d53_1" = 8
  measures "d52_1" diameter of A0
  measures "d53_1" diameter of A1
extrude "Extrude8'" cut sketch "Sketch7 (2)" against normal blind 46 contours E0 A0 | E0 A0 | A1 picked at (-12.249, -36.9652) picked at (-12.4627, -42.2784) bodies 14 in component "pipe-slider2"
extrude "Extrude10" cut sketch "Sketch1 (13)" along normal blind 5 contours L36 L37 L38 L39 L58 | L36 L37 L57 | L40 L41 L42 L43 L60 | L41 L42 L59 | L44 L45 L46 L50 L51 | L47 L48 L49 L52 L53 | L54 L55 L56 | L61 L62 L63 bodies 14 in component "pipe-slider2"
ref_plane "WorkPlane1" through (24, 0, -20) normal (1, 0, 0) x (0, 1, 0) in component "pipe-slider2"
sketch "Sketch9" plane through (24, 0, -20) normal (1, 0, 0) x (0, 1, 0) in component "pipe-slider2"
  line L0 (-2, -19.4868) -> (-2, 1)
  line L1 (-2, 1) -> (-4, 3)
  line L2 (2, -19.4868) -> (2, 1)
  line L3 (2, 1) -> (4, 3)
  line L4 (-45, 10) -> (-40, 15)
  line L5 (-40, 15) -> (-35, 10)
  line L6 (-35, 10) -> (-35, -19.4868)
  line L7 (-35, -19.4868) -> (-45, -19.4868)
  line L8 (-45, -19.4868) -> (-45, 10)
  line L9 (35, 10) -> (40, 15)
  line L10 (40, 15) -> (45, 10)
  line L11 (45, 10) -> (45, -19.5718)
  line L12 (45, -19.5718) -> (35, -19.5718)
  line L13 (35, -19.5718) -> (35, 10)
  line L14 (-32, -19.2) -> (-24.9423, -12.6544)
  line L15 (-24.9423, -12.6544) -> (-31.9999, -5.0446)
  line L16 (-31.9999, -5.0446) -> (-32, -19.2)
  line L17 (32, -19.5) -> (32, -5)
  line L18 (32, -5) -> (24.7296, -12.263)
  line L19 (24.7296, -12.263) -> (32, -19.5)
  line L20 (10.0346, -19.4868) -> (10.0346, -3.3896)
  line L21 (14, -7.5882) -> (14, -19.4868)
  line L22 (4, 3) -> (10.0346, -3.3896)
  line L23 (14, -7.5882) -> (25.2375, -19.4868)
  line L24 (25.2375, -19.4868) -> (14, -19.4868)
  line L25 (10.0346, -19.4868) -> (2, -19.4868)
  line L26 (-10, -3) -> (-10, -19.4868)
  line L27 (-15, -8) -> (-15, -19.4868)
  line L28 (-26.4868, -19.4868) -> (-15, -19.4868)
  line L29 (-10, -19.4868) -> (-2, -19.4868)
  line L30 (-4, 3) -> (-10, -3)
  line L31 (-15, -8) -> (-26.4868, -19.4868)
  constraint vertical L0
  constraint perpendicular L1 L30
  constraint perpendicular L0 L28
  constraint perpendicular L2 L28
  constraint parallel L3 L30
  constraint perpendicular L2 L24
  constraint parallel L4 L30
  constraint perpendicular L5 L30
  constraint perpendicular L6 L24
  constraint perpendicular L2 L7
  constraint perpendicular L7 L8
  constraint parallel L4 L9
  constraint perpendicular L4 L10
  constraint parallel L8 L11
  constraint perpendicular L8 L12
  constraint perpendicular L12 L13
  constraint perpendicular L14 L15
  constraint perpendicular L17 L24
  constraint coincident L20.start L24
  constraint perpendicular L20 L24
  constraint perpendicular L21 L24
  constraint collinear L22 L23
  constraint collinear L24 L25
  constraint coincident L26.end L28
  constraint perpendicular L26 L28
  constraint coincident L27.start L30
  constraint perpendicular L27 L28
  constraint collinear L28 L29
  constraint collinear L30 L31
extrude "Extrude11" cut sketch "Sketch9" against normal blind 5 bodies 14 in component "pipe-slider2"
chamfer "Chamfer2" distance 3 angle 45 8 edges at (19, -45, -24.7434) (19, 35, -24.7859) (5, 45, -24.773) (5, -35, -24.74) (19, 45, -24.7859) (19, -35, -24.7434) (5, 35, -24.773) (5, -45, -24.74) on bodies 14 in component "pipe-slider2"
extrude "Extrude12" add sketch "Sketch1 (13)" against normal blind 4 contours L4 L5 L6 L7 L29 A2 L31 L32 L33 L34 L35 | L29 A2 L31 L32 | A2 L33 L34 L35 | L36 L37 L38 L39 L58 | L36 L37 L57 L58 | L36 L37 L57 | L40 L41 L42 L43 L60 | L41 L42 L59 L60 | L41 L42 L59 | L44 L45 L46 L50 L51 | L47 L48 L49 L52 L53 | L54 L55 L56 | L61 L62 L63 bodies 14 in component "pipe-slider2"
extrude "Extrude13" add sketch "Sketch6 (2)" sketch "Sketch2 (4)" along normal blind 4 of sketch 2 bodies 14 in component "pipe-slider2"
chamfer "Chamfer3" distance 5 angle 45 4 edges at (0, -25.8094, -25.8094) (24, -25.8094, -25.8094) (24, 25.8094, -25.8094) (0, 25.8094, -25.8094) on bodies 14 in component "pipe-slider2"
chamfer "Chamfer4" distance 2 angle 45 4 edges at (-4, -50, -20) (28, -50, -20) (-4, 50, -20) (28, 50, -20) on bodies 14 in component "pipe-slider2"
component "pipe-d25mm" placed x (1, 0, 0) y (0, 1, 0) z (0, 0, 1) at (33.5624, 0, 0)
component "pipe-slider" placed x (1, 0, 0) y (0, 1, 0) z (0, 0, 1) at (0, 0, 0)
component "washer" placed x (1, 0, 0) y (0, 1, 0) z (0, 0, 1) at (0, 0, 0)
component "washer" placed x (1, 0, 0) y (0, 1, 0) z (0, 0, 1) at (0, 6.0104, 6.0104)
component "bearing8x22x7" placed x (1, 0, 0) y (0, 1, 0) z (0, 0, 1) at (0, 0, 0)
component "washer" placed x (1, 0, 0) y (0, 0, -1) z (0, 1, 0) at (0, 6.0104, -6.0104)
component "washer" placed x (1, 0, 0) y (0, 0, 1) z (0, -1, 0) at (0, -39.2444, -27.2236)
component "bearing8x22x7" placed x (1, 0, 0) y (0, 0, -1) z (0, 1, 0) at (0, 0, 0)
component "stud-30mm-d8mm" placed x (1, 0, 0) y (0, 1, 0) z (0, 0, 1) at (0, 0, 0)
component "pipe-slider" placed x (1, 0, 0) y (0, -1, 0) z (0, 0, -1) at (0, 0, 0.1848)
component "pipe-slider" placed x (1, 0, 0) y (0, 1, 0) z (0, 0, 1) at (-250, 0, 0)
component "pipe-slider" placed x (1, 0, 0) y (0, -1, 0) z (0, 0, -1) at (-250, 0, 0.1848)
component "frame-bottom" placed x (1, 0, 0) y (0, 1, 0) z (0, 0, 1) at (-100, 0, 0)
component "frame-top" placed x (1, 0, 0) y (0, -0.707107, -0.707107) z (0, 0.707107, -0.707107) at (-110, -36.8701, 126.6102)
component "cut-tool-12x12" placed x (1, 0, 0) y (0, 0.707107, -0.707107) z (0, 0.707107, 0.707107) at (0, -35.4558, 6.402)
component "pipe-to-frame-clump" placed x (1, 0, 0) y (0, 1, 0) z (0, 0, 1) at (-100, 0, 0)
component "pipe-to-frame-clump-insert" placed x (1, 0, 0) y (0, 1, 0) z (0, 0, 1) at (0, 0, 0)
component "pipe-to-frame-clump" placed x (1, 0, 0) y (0, 1, 0) z (0, 0, 1) at (-184, 0, 0)
component "pipe-to-frame-clump-insert" placed x (1, 0, 0) y (0, 1, 0) z (0, 0, 1) at (-84, 0, 0)
component "washer" placed x (1, 0, 0) y (0, -0.707107, -0.707107) z (0, 0.707107, -0.707107) at (-130, 45.5, -26)
component "washer" placed x (1, 0, 0) y (0, 0.707107, 0.707107) z (0, -0.707107, 0.707107) at (-130, -45.5, -17.5)
component "bearing8x22x7" placed x (1, 0, 0) y (0, -0.707107, -0.707107) z (0, 0.707107, -0.707107) at (-130, 45.5, -26)
component "nut-m8" placed x (1, 0, 0) y (0, 1, 0) z (0, 0, 1) at (0, 0, 0)
component "bearing8x22x7" placed x (1, 0, 0) y (0, -0.707107, -0.707107) z (0, 0.707107, -0.707107) at (-130, 1.5, -26)
component "nut-m8" placed x (1, 0, 0) y (0, 1, 0) z (0, 0, 1) at (0, 44, 0)
component "corner" placed x (1, 0, 0) y (0, 1, 0) z (0, 0, 1) at (100, 0, 0)
component "corner" placed x (-1, 0, 0) y (0, -1, 0) z (0, 0, 1) at (-270, -0.0082, 0)
component "pipe-slider2" placed x (1, 0, 0) y (0, 1, 0) z (0, 0, 1) at (0, 0, 0)
